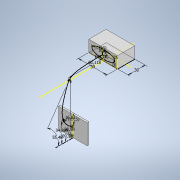
# Autodesk Inventor part: Verbindung_Motor_Servo
Saved by Autodesk Inventor 2021 (Build 250183000, 183)
## iProperties
Created: 2021-01-04
Part Number: Verbindung_Motor_Servo
Material: Generisch
Document SubType Name: Modeling
Designer: Ctroi
Density: 1 g/cm^3
Appearance: Vorgabe
Mass: 91.5133 g
Surface Area: 197.408 cm^2
Volume: 91.5133 cm^3
Author: Ctroi
## iProperties of the stored document _3D-Druck.ipt
Created: 2021-01-04
Part Number: _3D-Druck
Material: Generisch
Document SubType Name: Modeling
Designer: Ctroi
Density: 1 g/cm^3
Appearance: Vorgabe
Author: Ctroi
Autodesk Inventor part; units mm, degrees
ref_plane "YZ Plane" through (0, 0, 0) normal (1, 0, 0) x (0, 1, 0)
ref_plane "XZ Plane" through (0, 0, 0) normal (0, 1, 0) x (-1, 0, 0)
sketch "Skizze1" plane through (0, 0, 0) normal (0, 1, 0) x (-1, 0, 0)
  line L0 (25, -15) -> (-25, -15)
  line L1 (-25, -15) -> (-25, 15)
  line L2 (-25, 15) -> (25, 15)
  line L3 (25, 15) -> (25, -15)
  line L4 (35, 0) -> (-35, 0) projected
  line L5 (0, -38.6491) -> (0, 126.8947) projected
  point P0 (0, 0)
  dimension "d0" = 50
  dimension "d1" = 30
  constraints: 8 end point, 2 parallel, 1 horizontal, 1 perpendicular, 2 other
  measures "d0" distance of L1.end L2.end
  measures "d1" distance of L0.end L1.end
extrude "Extrusion1" add sketch "Skizze1" along normal blind 20
ref_plane "Arbeitsebene1" through (-25, 0, 68) normal (0, 0, 1) x (1, 0, 0)
sketch "Skizze10" plane through (-25, 0, 68) normal (0, 0, 1) x (1, 0, 0)
  line L0 (50, -55) -> (0, -55)
  line L1 (0, -55) -> (0, -90)
  line L2 (0, -90) -> (50, -90)
  line L3 (50, -90) -> (50, -55)
  line L4 (0, 0) -> (50, 0) projected
  line L5 (25, -112) -> (25, 42) projected
  point P0 (25, 0)
  dimension "d44" = 50
  dimension "d45" = 35
  dimension "d46" = 55
  constraints: 8 end point, 2 parallel, 1 horizontal, 1 perpendicular, 1 other
  measures "d44" distance of L2.end L1.end
  measures "d45" distance of L1.end L0.end
  measures "d46" distance between parallel lines of L4 L0
extrude "Extrusion7" add sketch "Skizze10" against normal blind 3
sketch "Skizze11" plane through (-25, 0, 15) normal (0, 0, 1) x (1, 0, 0)
  ellipse E0 centre (25, 10) end of major axis (45, 10) minor radius 7.5
  line L0 (0, 0) -> (50, 0) projected
  line L1 (50, 0) -> (50, 20) projected
  point P0 (25, 0)
  dimension "d49" = 10
  dimension "d50" = 25
  dimension "d51" = 20
  dimension "d52" = 7.5
  constraints: 1 centre point, 1 other
  measures "d49" distance from line of L0 E0.centre
  measures "d50" distance from line of L1 E0.centre
  measures "d51" diameter of E0
sketch "Skizze12" plane through (0, 0, 0) normal (1, 0, 0) x (0, 1, 0)
  line L0 (0, 15) -> (20, 15) projected
  line L1 (-55, 68) -> (-90, 68) projected
  spline S0 degree 4 poles (10, 15) (9.9748, 21.2064) (9.8777, 76.735) (3.1904, 71.0475) (-60.3346, 101.6715) (-72.933, 67.6671) (-72.5, 68) knots 0 0 0 0 0 0.382337 0.571486 1 1 1 1 1
  line L2 (-90, 68) -> (-90, 98.8668)
  line L3 (-90, 68) -> (-90, 65) projected
  line L4 (7.9908, 69.6224) -> (-7.9908, 80.6145) construction
  arc A0 (4.9597, 69.8562) -> (-6.6882, 77.8676) centre (-9.7151, 60.9936) ccw construction
  line L5 (-38.6667, 91.0844) -> (-71.5552, 78.5361) construction
  arc A1 (-42.1089, 86.8611) -> (-66.1746, 77.679) centre (-43.7525, 55.0405) ccw construction
  line L6 (10.0269, 8.386) -> (9.9731, 21.614) construction
  arc A2 (10.0019, 20.2911) -> (10.0449, 9.7091) centre (607.2373, 17.4262) ccw construction
  line L7 (-90, 68) -> (-90, 65) projected
  point P0 (0, 0)
  point P1 (0, 75.1185)
  point P2 (-55.1109, 84.8102)
  dimension "d54" = 10
  dimension "d59" = 0.409
  dimension "d60" = 0.5998
  dimension "d61" = 1.0884
  dimension "d62" = 20.884
  dimension "d63" = 69.116
  dimension "d64" = 16.8102
  dimension "d65" = 34.8891
  dimension "d66" = 17.5
  dimension "d67" = 60.1185
  dimension "d68" = 90
  dimension "d69" = 55.48
  dimension "d70" = 9.9999
  dimension "d71" = 89.767
  constraints: 8 end point, 8 midpoint, 3 centre point, 3 point on circle, 1 vertical, 10 other
  measures "d54" distance of L0.end point (10, 15)
  measures "d62" angle of L1 L5
  measures "d63" angle of L3 L5
  measures "d64" distance from line of L1 point (-55.111, 84.81)
  measures "d65" horizontal distance of L1.end point (-55.111, 84.81)
  measures "d66" distance of L1.start point (-72.5, 68)
  measures "d67" distance from line of L0 point (0, 75.118)
  measures "d68" distance from line of L7 point (0, 75.118)
  measures "d69" angle of L3 L4
  measures "d70" distance from line of L0.start L6
  measures "d71" angle of L0 L6
